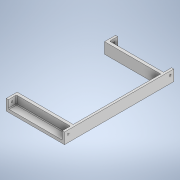
# Autodesk Inventor part: leg_8u
Saved by Autodesk Inventor 2021.3 (Build 253353010, 353A)
## iProperties
Created: 2021-10-20
Part Number: leg_8u
Material: Generic
Document SubType Name: Modeling
Designer: jesse
Density: 1 g/cm^3
Appearance: Default
Author: jesse
Autodesk Inventor part; units mm, degrees
ref_plane "YZ Plane" through (0, 0, 0) normal (1, 0, 0) x (0, 1, 0)
ref_plane "XZ Plane" through (0, 0, 0) normal (0, 1, 0) x (-1, 0, 0)
ref_plane "XY Plane" through (0, 0, 0) normal (0, 0, 1) x (1, 0, 0)
sketch "Sketch1" plane through (0, 0, 0) normal (0, 1, 0) x (-1, 0, 0)
  line L0 (41.8301, 96.0131) -> (-38.1699, 96.0131)
  line L1 (-38.1699, 96.0131) -> (-38.1699, -53.9869)
  line L2 (-38.1699, -53.9869) -> (41.8301, -53.9869)
  line L3 (41.8301, -53.9869) -> (41.8301, 96.0131)
  line L4 (41.8301, 81.0131) -> (-35.1699, 81.0131)
  line L5 (-35.1699, 81.0131) -> (-35.1699, -38.9869)
  line L6 (-35.1699, -38.9869) -> (41.8301, -38.9869)
  line L7 (41.8301, -38.9869) -> (41.8301, 81.0131)
  point P0 (0, 0)
  dimension "d0" = 80
  dimension "d1" = 150
  dimension "d2" = 15
  dimension "d3" = 15
  dimension "d4" = 3
  constraints: 16 end point, 4 parallel, 2 horizontal, 2 perpendicular, 1 point on line
  measures "d0" distance of L1.end L2.end
  measures "d1" distance of L2.end L0.start
  measures "d2" distance between parallel lines of L4 L0
  measures "d3" distance between parallel lines of L2 L6
  measures "d4" distance between parallel lines of L1 L5
extrude "Extrusion1" add sketch "Sketch1" along normal blind 15 contours L3 L4 L5 L6 L2 L1 L0
sketch "Sketch2" plane through (0, 15, 0) normal (0, 1, 0) x (1, 0, 0)
  line L0 (-41.8301, -96.0131) -> (38.1699, -96.0131) projected
  line L1 (-38.8301, -96.0131) -> (35.1699, -96.0131)
  line L2 (35.1699, -96.0131) -> (35.1699, -85.0131)
  line L3 (35.1699, -85.0131) -> (-38.8301, -85.0131)
  line L4 (-38.8301, -85.0131) -> (-38.8301, -96.0131)
  line L5 (38.1699, 53.9869) -> (-41.8301, 53.9869) projected
  line L6 (-38.8301, 53.9869) -> (35.1699, 53.9869)
  line L7 (35.1699, 53.9869) -> (35.1699, 42.9869)
  line L8 (35.1699, 42.9869) -> (-38.8301, 42.9869)
  line L9 (-38.8301, 42.9869) -> (-38.8301, 53.9869)
  line L10 (35.1699, -81.0131) -> (-41.8301, -81.0131) projected
  line L11 (-41.8301, 38.9869) -> (35.1699, 38.9869) projected
  line L12 (-41.8301, 53.9869) -> (-41.8301, 38.9869) projected
  point P0 (0, 0)
  point P1 (35.1699, -96.0131)
  dimension "d7" = 4
  dimension "d8" = 4
  dimension "d9" = 3
  constraints: 16 end point, 4 parallel, 4 point on line, 2 horizontal, 2 perpendicular
  measures "d7" distance between parallel lines of L10 L3
  measures "d8" distance between parallel lines of L8 L11
  measures "d9" distance between parallel lines of L12 L9
extrude "Extrusion2" cut sketch "Sketch2" against normal blind 11
sketch "Sketch3" plane through (-41.8301, 0, -53.9869) normal (-1, 0, 0) x (0, 0, 1)
  circle A0 centre (5, 10) radius 1.3
  circle A1 centre (145, 10) radius 1.3
  line L0 (11, 15) -> (11, 4) projected
  line L1 (11, 4) -> (0, 4) projected
  line L2 (139, 15) -> (139, 4) projected
  line L3 (150, 4) -> (139, 4) projected
  point P0 (53.9869, 0)
  dimension "d12" = 2.6
  dimension "d13" = 2.6
  dimension "d14" = 6
  dimension "d15" = 6
  dimension "d16" = 6
  dimension "d17" = 6
  constraints: 2 centre point
  measures "d12" diameter of A0
  measures "d13" diameter of A1
  measures "d14" distance from line of L0 A0.centre
  measures "d15" distance from line of L1 A0.centre
  measures "d16" distance from line of L2 A1.centre
  measures "d17" distance from line of L3 A1.centre
extrude "Extrusion3" cut sketch "Sketch3" against normal through all
fillet "Fillet1" radius 1 5 edges at (-1.8301, 4, -42.9869) (-38.8301, 9.5, -42.9869) (-38.8301, 4, -48.4869) (35.1699, 4, -48.4869) (35.1699, 9.5, -42.9869)
fillet "Fillet2" radius 1 5 edges at (-38.8301, 9.5, 85.0131) (-38.8301, 4, 90.5131) (-1.8301, 4, 85.0131) (35.1699, 9.5, 85.0131) (35.1699, 4, 90.5131)
body "Solid1"
